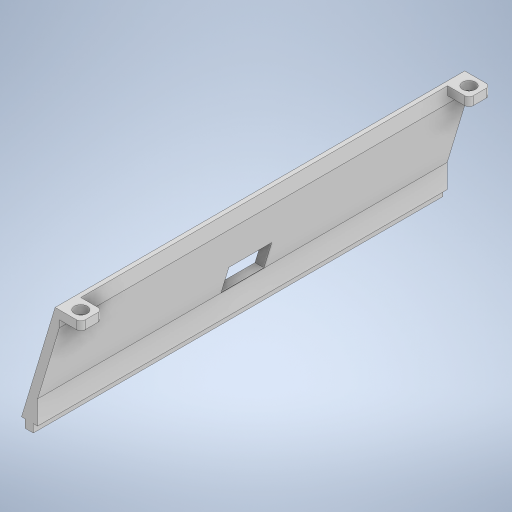
# Autodesk Inventor part: Přední rampa POKUS
Saved by Autodesk Inventor 2024 (Build 280153000, 153)
## iProperties
Created: 2023-05-12
Part Number: Přední rampa POKUS
Material: Všeobecné
Document SubType Name: Modeling
Designer: jaryj
Density: 1 g/cm^3
Appearance: Výchozí
Author: jaryj
Autodesk Inventor part; units mm, degrees
ref_plane "YZ Plane" through (0, 0, 0) normal (1, 0, 0) x (0, 1, 0)
ref_plane "XZ Plane" through (0, 0, 0) normal (0, 1, 0) x (-1, 0, 0)
ref_plane "XY Plane" through (0, 0, 0) normal (0, 0, 1) x (1, 0, 0)
sketch "Náčrt1" plane through (0, 0, 0) normal (0, 0, 1) x (1, 0, 0)
  line L0 (0, 0) -> (7.8261, 26)
  line L1 (0, 0) -> (0.8442, 0)
  line L2 (0.8442, 0) -> (0.8442, -1.9)
  line L3 (0.8442, -1.9) -> (2.7442, -1.9)
  line L4 (2.7442, -1.9) -> (2.7442, 0)
  line L5 (2.7442, 0) -> (3.7442, 0)
  line L6 (3.7442, 0) -> (3.7442, 5.5)
  line L7 (3.7442, 5.5) -> (8.8261, 22.3833)
  line L8 (8.8261, 22.3833) -> (8.8261, 26)
  line L9 (8.8261, 26) -> (7.8261, 26)
  line L10 (3.7442, 0) -> (18.7442, 0) construction
  line L11 (0, 0) -> (-1.1739, -3.9) construction
  dimension "d0" = 1.9
  dimension "d1" = 1.9
  dimension "d2" = 1
  dimension "d4" = 5.5
  dimension "d5" = 2
  dimension "d6" = 1
  dimension "d7" = 26
  dimension "d10" = 15
  dimension "d27" = 10
  dimension "d28" = 2
  constraints: 24 end point, 5 perpendicular, 3 point on line, 2 horizontal, 1 parallel, 1 vertical
  measures "d0" distance of L2.end L3.end
  measures "d1" distance of L3.end L4.end
  measures "d2" distance of L4.end L5.end
  measures "d4" distance of L5.end L6.end
  measures "d5" distance between parallel lines of L0 L7
  measures "d6" distance of L8.end L0.end
  measures "d7" distance between parallel lines of L5 L9
  measures "d10" distance of L5.end L10.end
  measures "d27" horizontal distance of L8.end L11.end
  measures "d28" vertical distance of L2.end L11.end
extrude "Vysunutí1" add sketch "Náčrt1" along normal blind 47.75
sketch "Náčrt2" plane through (7.8261, 26, 0) normal (0, 1, 0) x (1, 0, 0)
  line L0 (1, 0) -> (1, -47.75) projected
  line L1 (1, 0) -> (6, 0)
  line L2 (6, 0) -> (6, -5)
  line L3 (6, -5) -> (1, -5)
  line L4 (1, -5) -> (1, 0)
  point P0 (-7.8261, 0)
  point P1 (1, -5)
  dimension "d13" = 5
  dimension "d14" = 5
  constraints: 8 end point, 2 parallel, 1 horizontal, 1 perpendicular
  measures "d13" distance of L2.end L3.end
  measures "d14" distance of L1.end L2.end
extrude "Vysunutí2" add sketch "Náčrt2" against normal blind 2
sketch "Náčrt4" plane through (8.8261, 22.3833, 47.75) normal (1, 0, 0) x (0, 0, -1)
  line L0 (0, 3.6167) -> (0, -22.3833) projected
  line L1 (0, -10.7833) -> (5, -10.7833)
  line L2 (5, -10.7833) -> (5, -16.7833)
  line L3 (5, -16.7833) -> (0, -16.7833)
  line L4 (0, -16.7833) -> (0, -10.7833)
  line L5 (47.75, -24.2833) -> (0, -24.2833) projected
  point P0 (47.75, -22.3833)
  point P1 (0, -16.7833)
  dimension "d29" = 7.5
  dimension "d30" = 6
  dimension "d31" = 5
  constraints: 8 end point, 2 parallel, 1 horizontal, 1 perpendicular, 1 point on line
  measures "d29" distance between parallel lines of L3 L5
  measures "d30" distance of L1.end L2.end
  measures "d31" distance of L1.start L1.end
extrude "Vysunutí3" cut sketch "Náčrt4" against normal through all
sketch "Náčrt3" plane through (7.8261, 26, 47.75) normal (0, 1, 0) x (1, 0, 0)
  line L0 (1, 42.75) -> (6, 42.75) projected
  line L1 (6, 42.75) -> (6, 47.75) projected
  point P0 (-7.8261, 47.75)
  point P1 (3.5, 45.25)
  dimension "d17" = 2.5
  dimension "d25" = 2.5
  measures "d17" distance from line of L0 point (3.5, 45.25)
  measures "d25" distance from line of L1 point (3.5, 45.25)
hole "Díra1" at (11.3261, 26, 2.5) direction (0, -1, 0) diameter 3 depth 6
fillet "Zaoblení1" radius 1 2 edges at (13.8261, 25, 5) (13.8261, 25, 0)
mirror "Zrcadlit1" about plane through (4.413, 12.05, 47.75) normal (0, 0, 1)
